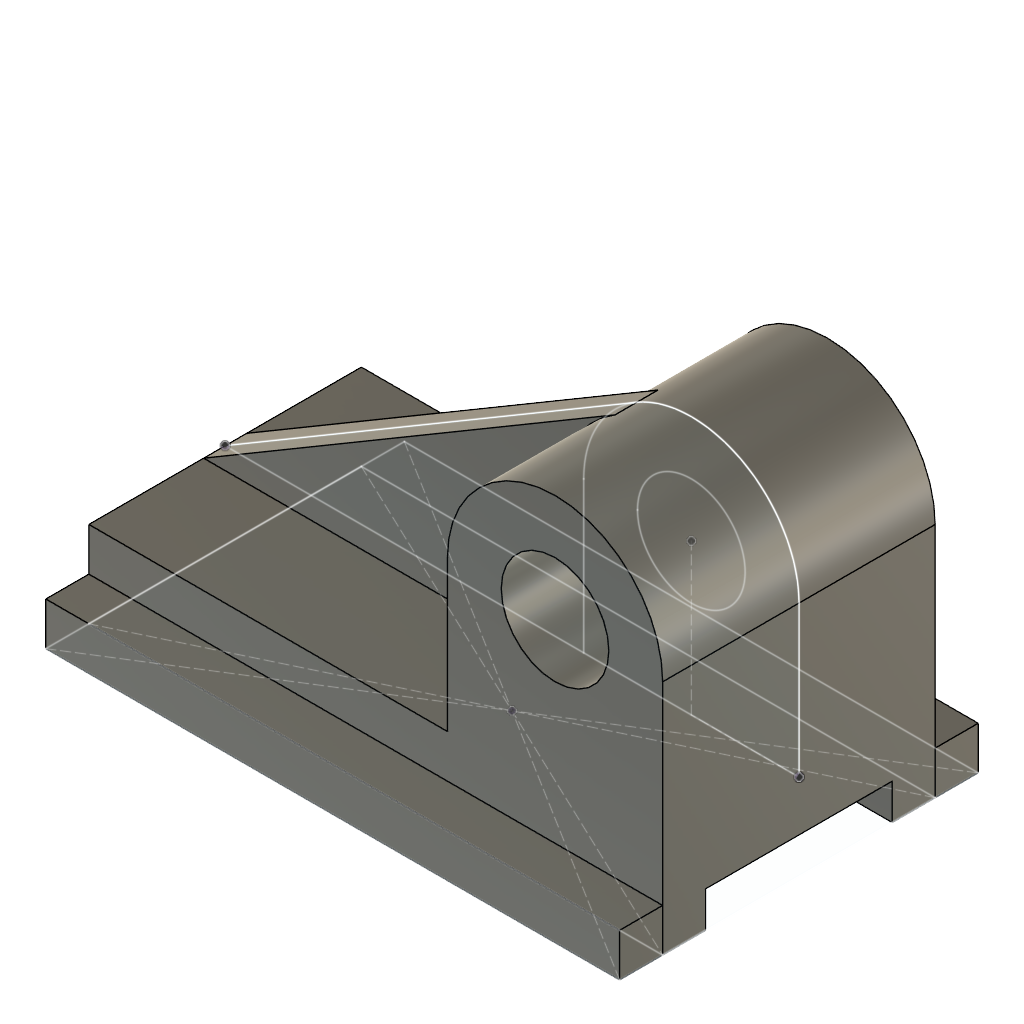
fusion exercise 4 (Autodesk Fusion 360 design; units mm, degrees)
part number: 2026-09-22-16-44-19-079
Autodesk Fusion 360 part; units mm, degrees
sketch "Sketch1" plane through (0, 0, 0) normal (0, 0, 1) x (1, 0, 0)
  line L0 (80, -50) -> (-80, -50)
  line L1 (-80, -50) -> (-80, 50)
  line L2 (-80, 50) -> (80, 50)
  line L3 (80, 50) -> (80, -50)
  line L4 (80, -50) -> (-80, 50) construction
  line L5 (-80, -50) -> (80, 50) construction
  line L6 (80, 38) -> (-80, 38)
  line L7 (-80, 38) -> (-80, -38)
  line L8 (-80, -38) -> (80, -38)
  line L9 (80, -38) -> (80, 38)
  line L10 (80, 38) -> (-80, -38) construction
  line L11 (-80, 38) -> (80, -38) construction
  dimension "d1" = 160
  dimension "d2" = 100
  dimension "d3" = 160
  dimension "d4" = 76
  constraint horizontal L0
  constraint perpendicular L0 L1
  constraint parallel L0 L2
  constraint parallel L1 L3
  constraint coincident L4 origin
  constraint coincident L5 origin
  constraint horizontal L6
  constraint perpendicular L6 L7
  constraint parallel L6 L8
  constraint parallel L7 L9
  constraint coincident L10 origin
  constraint coincident L11 origin
  measures "d1" distance of L1.end L2.end
  measures "d2" distance of L0.end L1.end
  measures "d3" distance of L7.end L8.end
  measures "d4" distance of L6.end L7.end
extrude "Extrude1" add sketch "Sketch1" along normal blind 12 contours L0 L1 L3 L8 | L1 L2 L3 L6 makes body 1 at (26.6667, 38, 4) makes body 2 at (26.6667, -50, 4)
extrude "Extrude2" add sketch "Sketch1" along normal blind 24 separate body contours L1 L3 L6 L7 L8 L9 makes body 3
sketch "Sketch2" plane through (-80, 0, 0) normal (-1, 0, 0) x (0, -1, 0)
  line L0 (-38, 0) -> (38, 0)
  line L1 (38, 0) -> (38, 24)
  line L2 (38, 24) -> (-38, 24)
  line L3 (-38, 24) -> (-38, 0)
  line L4 (26, 10) -> (-26, 10)
  line L5 (-26, 10) -> (-26, -10)
  line L6 (-26, -10) -> (26, -10)
  line L7 (26, -10) -> (26, 10)
  line L8 (26, 10) -> (-26, -10) construction
  line L9 (-26, 10) -> (26, -10) construction
  dimension "d9" = 52
  dimension "d10" = 20
  constraint horizontal L4
  constraint perpendicular L4 L5
  constraint parallel L4 L6
  constraint parallel L5 L7
  constraint coincident L8 origin
  constraint coincident L9 origin
  measures "d9" distance of L5.end L6.end
  measures "d10" distance of L4.end L5.end
extrude "Extrude3" cut sketch "Sketch2" against normal up to surface (160 mm away) contours L0 L4 L5 L7 bodies 3
ref_plane "WorkPlane1" through (0, 0, 6) normal (0, -1, 0) x (1, 0, 0)
sketch "Sketch3" plane through (0, 0, 0) normal (0, -1, 0) x (-1, 0, 0)
  line L0 (-80, -24) -> (-50, -24) construction
  line L1 (-50, -24) -> (-50, -66) construction
  circle A0 centre (-50, -66) radius 15
  line L2 (-80, -66) -> (-80, -24)
  line L3 (-20, -66) -> (-20, -24)
  line L4 (80, -24) -> (-34.7335, -91.825)
  line L5 (80, -24) -> (-80, -24)
  arc A1 (-80, -66) -> (-20, -66) centre (-50, -66) ccw
  point P0 (80, -24)
  point P1 (-80, -24)
  dimension "d13" = 30
  dimension "d14" = 42
  dimension "d15" = 60
  dimension "d16" = 30
  constraint horizontal L0
  constraint perpendicular L0 L1
  constraint coincident L1.end A0.centre
  constraint perpendicular L0 L3
  constraint coincident L4.end A1
  constraint tangent L4 A1
  constraint parallel L0 L5
  constraint coincident P0 L4.start
  constraint coincident L3.end L5
  constraint coincident L0.start L2.end
  constraint tangent L3 A1
  constraint tangent L2 A1
  measures "d13" distance of L0.start L0.end
  measures "d14" distance of L0.end L1.end
  measures "d15" diameter of A1
  measures "d16" diameter of A0
extrude "Extrude4" add sketch "Sketch3" along normal mid plane 76 contours L2 L3 L5 A1 bodies 3
extrude "Extrude5" add sketch "Sketch3" along normal mid plane 12 contours L3 L4 L5 A1 bodies 3
